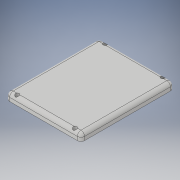
# Autodesk Inventor part: top
Saved by Autodesk Inventor 2017 (Build 210142000, 142)
## iProperties
Created: 2018-05-31
Part Number: top
Material: Generic
Document SubType Name: Modeling
Designer: sinner
Density: 1 g/cm^3
Appearance: Default
Author: sinner
Autodesk Inventor part; units mm, degrees
ref_plane "YZ Plane" through (0, 0, 0) normal (1, 0, 0) x (0, 1, 0)
ref_plane "XZ Plane" through (0, 0, 0) normal (0, 1, 0) x (-1, 0, 0)
ref_plane "XY Plane" through (0, 0, 0) normal (0, 0, 1) x (1, 0, 0)
sketch "Sketch1" plane through (0, 0, 0) normal (0, 1, 0) x (-1, 0, 0)
  line L0 (0, 0) -> (66.04, 0)
  line L1 (66.04, 0) -> (66.04, -81.915)
  line L2 (66.04, -81.915) -> (0, -81.915)
  line L3 (0, -81.915) -> (0, 0)
  dimension "d0" = 66.04
  dimension "d1" = 81.915
  constraints: 8 end point, 2 parallel, 1 horizontal, 1 perpendicular
  measures "d0" distance of L1.end L2.end
  measures "d1" distance of L2.end L0.start
extrude "Extrusion1" add sketch "Sketch1" along normal blind 6.35
fillet "Fillet1" radius 3.175 4 edges at (0, 3.175, 0) (-66.04, 3.175, 0) (0, 3.175, -81.915) (-66.04, 3.175, -81.915)
fillet "Fillet2" radius 3.175 8 edges at (-0.9299, 6.35, -80.9851) (-33.02, 6.35, -81.915) (-65.1101, 6.35, -80.9851) (-66.04, 6.35, -40.9575) (-65.1101, 6.35, -0.9299) (-33.02, 6.35, 0) (-0.9299, 6.35, -0.9299) (0, 6.35, -40.9575)
sketch "Sketch2" plane through (0, 6.35, 0) normal (0, 1, 0) x (1, 0, 0)
  line L0 (0, 0) -> (0, 23.0418) construction
  line L1 (0, 78.74) -> (0, 3.175) projected
  line L2 (0, 0) -> (-15.3745, 0) construction
  line L3 (-3.175, 0) -> (-62.865, 0) projected
  line L4 (0, 2.3813) -> (-36.1213, 2.3813) construction
  line L5 (-33.02, 0) -> (-33.02, 49.3607) construction
  circle A0 centre (-7.62, 2.3813) radius 1.632
  line L6 (-3.175, 78.74) -> (-3.175, 3.175) projected
  line L7 (-3.175, 40.9575) -> (-28.1102, 40.9575) construction
  circle A1 centre (-58.42, 2.3813) radius 1.632
  circle A2 centre (-7.62, 79.5337) radius 1.632
  circle A3 centre (-58.42, 79.5337) radius 1.632
  dimension "d6" = 2.3813
  dimension "d7" = 3.2639
  dimension "d8" = 25.4
  constraints: 10 end point, 4 centre point, 4 point on line, 3 symmetric about line, 2 horizontal, 2 midpoint, 1 vertical, 3 other
  measures "d6" distance between parallel lines of L2 L4
  measures "d7" diameter of A0
  measures "d8" distance from line of L5 A0.centre
extrude "Extrusion2" cut sketch "Sketch2" against normal blind 6.35
body "Solid1"
